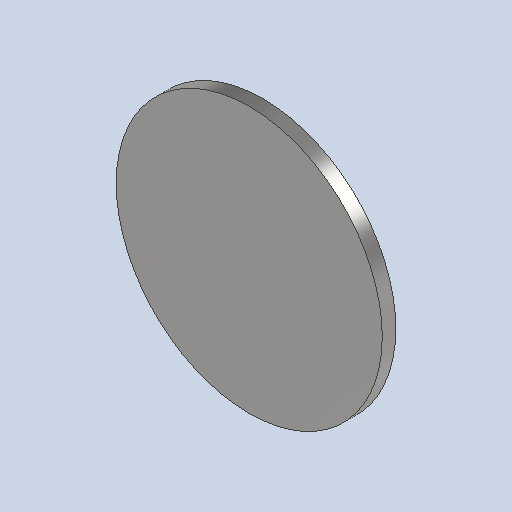
# Autodesk Inventor part: NDM 4.0.5 base plate
Saved by Autodesk Inventor 2025 (Build 290162010, 162A)
## iProperties
Created: 2023-07-02
Part Number: NDM 4.0.5 base plate
Material: Stainless Steel
Document SubType Name: Sheet Metal
Designer: user
Density: 8 g/cm^3
Appearance: Semi-Polished
Stock Number: NDM 12.1 base plate
Flat Pattern Width: 5.9 cm
Flat Pattern Length: 5.9 cm
Flat Pattern Area: 34.81 cm^2
Sheet Metal Rule: Default
Sheet Metal Width: 59,000 mm
Sheet Metal Length: 59,000 mm
Sheet Metal Area: 3481,000 mm^2
Description: лист 3mm
Author: user
Revision Number: 1
Autodesk Inventor part; units mm, degrees
ref_plane "YZ Plane" through (0, 0, 0) normal (1, 0, 0) x (0, 1, 0)
ref_plane "XZ Plane" through (0, 0, 0) normal (0, 1, 0) x (-1, 0, 0)
ref_plane "XY Plane" through (0, 0, 0) normal (0, 0, 1) x (1, 0, 0)
sketch "Sketch1" plane through (0, 0, 0) normal (0, 0, 1) x (1, 0, 0)
  circle A0 centre (0, 0) radius 29.5
  dimension "d0" = 59
  constraints: 1 centre point, 1 coincident
  measures "d0" diameter of A0
extrude "Plate1" add sketch "Sketch1" along normal blind 3
equation "\"d3\" = Thickness"
equation "\"BendRadius\" = Thickness"
equation "\"BendReliefWidth\" = Thickness"
equation "\"BendReliefDepth\" = 0.5 * Thickness"
equation "\"CornerReliefSize\" = 4 * Thickness"
equation "\"MinimumRemnant\" = 2 * Thickness"
equation "\"TransitionRadius\" = BendRadius"
equation "\"JacobiRadiusSize\" = BendRadius"
equation "\"GapSize\" = Thickness"
equation "\"Thickness\" = 3"
body "Solid2"
